Autodesk Inventor part; units mm, degrees
(part 3 of 6)
  spline S504 degree 2 poles (-98.2003, 62.4281) (-98.3407, 62.5686) (-98.4987, 62.6915) knots 0 0 0 1 1 1
  spline S505 degree 2 poles (-71.4426, 63.5518) (-71.4426, 63.9557) (-70.8807, 64.5) (-70.4944, 64.5) knots 0 0 0 1 2 2 2
  spline S506 degree 2 poles (-70.4944, 64.5) (-70.0906, 64.5) (-69.5287, 63.9557) (-69.5287, 63.5518) knots 0 0 0 1 2 2 2
  line L659 (-69.5287, 63.5518) -> (-69.5287, 54.9657)
  line L660 (-69.5287, 54.9657) -> (-63.8222, 54.9657)
  line L661 (-63.8222, 54.9657) -> (-63.8222, 63.5518)
  spline S507 degree 2 poles (-63.8222, 63.5518) (-63.8222, 63.9557) (-63.2603, 64.5) (-62.8565, 64.5) knots 0 0 0 1 2 2 2
  spline S508 degree 2 poles (-62.8565, 64.5) (-62.4702, 64.5) (-61.9083, 63.9557) (-61.9083, 63.5518) knots 0 0 0 1 2 2 2
  line L662 (-61.9083, 63.5518) -> (-61.9083, 44.4482)
  spline S509 degree 2 poles (-61.9083, 44.4482) (-61.9083, 44.0619) (-62.4702, 43.5) (-62.8565, 43.5) knots 0 0 0 1 2 2 2
  spline S510 degree 2 poles (-62.8565, 43.5) (-63.2603, 43.5) (-63.8222, 44.0619) (-63.8222, 44.4482) knots 0 0 0 1 2 2 2
  line L663 (-63.8222, 44.4482) -> (-63.8222, 53.0518)
  line L664 (-63.8222, 53.0518) -> (-69.5287, 53.0518)
  line L665 (-69.5287, 53.0518) -> (-69.5287, 44.4482)
  spline S511 degree 2 poles (-69.5287, 44.4482) (-69.5287, 44.0619) (-70.0906, 43.5) (-70.4944, 43.5) knots 0 0 0 1 2 2 2
  spline S512 degree 2 poles (-70.4944, 43.5) (-70.8807, 43.5) (-71.4426, 44.0619) (-71.4426, 44.4482) knots 0 0 0 1 2 2 2
  line L666 (-71.4426, 44.4482) -> (-71.4426, 63.5518)
  spline S513 degree 2 poles (-33.3246, 49.8211) (-32.9383, 49.8211) (-32.3764, 49.2592) (-32.3764, 48.8554) knots 0 0 0 1 2 2 2
  spline S514 degree 2 poles (-32.3764, 48.8554) (-32.3764, 48.4691) (-32.9383, 47.9072) (-33.3246, 47.9072) knots 0 0 0 1 2 2 2
  line L667 (-33.3246, 47.9072) -> (-36.5026, 47.9072)
  line L668 (-36.5026, 47.9072) -> (-37.4684, 44.2901)
  spline S515 degree 2 poles (-37.4684, 44.2901) (-37.5562, 43.9916) (-37.7493, 43.7809) knots 0 0 0 1 1 1
  spline S516 degree 2 poles (-37.7493, 43.7809) (-38.0302, 43.5) (-38.4165, 43.5) knots 0 0 0 1 1 1
  spline S517 degree 2 poles (-38.4165, 43.5) (-38.8204, 43.5) (-39.3822, 44.0619) (-39.3822, 44.4482) knots 0 0 0 1 2 2 2
  spline S518 degree 2 poles (-39.3822, 44.4482) (-39.3822, 44.5711) (-39.3647, 44.6589) knots 0 0 0 1 1 1
  line L669 (-39.3647, 44.6589) -> (-34.2727, 63.6572)
  spline S519 degree 2 poles (-34.2727, 63.6572) (-34.2025, 63.9732) (-33.9918, 64.2015) knots 0 0 0 1 1 1
  spline S520 degree 2 poles (-33.9918, 64.2015) (-33.7108, 64.5) (-33.3246, 64.5) knots 0 0 0 1 1 1
  spline S521 degree 2 poles (-33.3246, 64.5) (-32.9383, 64.5) (-32.6398, 64.2015) knots 0 0 0 1 1 1
  spline S522 degree 2 poles (-32.6398, 64.2015) (-32.4642, 63.9732) (-32.394, 63.6572) knots 0 0 0 1 1 1
  line L670 (-32.394, 63.6572) -> (-27.302, 44.6589)
  spline S523 degree 2 poles (-27.302, 44.6589) (-27.2844, 44.5711) (-27.2844, 44.4482) knots 0 0 0 1 1 1
  spline S524 degree 2 poles (-27.2844, 44.4482) (-27.2844, 44.0619) (-27.8463, 43.5) (-28.2326, 43.5) knots 0 0 0 1 2 2 2
  spline S525 degree 2 poles (-28.2326, 43.5) (-28.6364, 43.5) (-28.8998, 43.7809) knots 0 0 0 1 1 1
  spline S526 degree 2 poles (-28.8998, 43.7809) (-29.1105, 43.9916) (-29.1983, 44.2901) knots 0 0 0 1 1 1
  line L671 (-29.1983, 44.2901) -> (-33.3246, 59.7943)
  line L672 (-33.3246, 59.7943) -> (-35.9935, 49.8211)
  line L673 (-35.9935, 49.8211) -> (-33.3246, 49.8211)
  spline S527 degree 2 poles (-4.4511, 63.8503) (-4.4511, 64.2542) (-3.8892, 64.8161) (-3.5029, 64.8161) knots 0 0 0 1 2 2 2
  spline S528 degree 2 poles (-3.5029, 64.8161) (-3.0991, 64.8161) (-2.5372, 64.2542) (-2.5372, 63.8503) knots 0 0 0 1 2 2 2
  line L674 (-2.5372, 63.8503) -> (-2.5372, 47.9599)
  spline S529 degree 2 poles (-2.5372, 47.9599) (-2.5372, 46.9064) (-1.0447, 45.4139) (0.0088, 45.4139) knots 0 0 0 1 2 2 2
  spline S530 degree 2 poles (0.0088, 45.4139) (1.0623, 45.4139) (2.5548, 46.9064) (2.5548, 47.9599) knots 0 0 0 1 2 2 2
  line L675 (2.5548, 47.9599) -> (2.5548, 63.8503)
  spline S531 degree 2 poles (2.5548, 63.8503) (2.5548, 64.2542) (3.0991, 64.8161) (3.5029, 64.8161) knots 0 0 0 1 2 2 2
  spline S532 degree 2 poles (3.5029, 64.8161) (3.9068, 64.8161) (4.4686, 64.2542) (4.4686, 63.8503) knots 0 0 0 1 2 2 2
  line L676 (4.4686, 63.8503) -> (4.4686, 47.9599)
  spline S533 degree 2 poles (4.4686, 47.9599) (4.4686, 46.1162) (1.8524, 43.5) (0.0088, 43.5) knots 0 0 0 1 2 2 2
  spline S534 degree 2 poles (0.0088, 43.5) (-1.8349, 43.5) (-4.4511, 46.1162) (-4.4511, 47.9599) knots 0 0 0 1 2 2 2
  line L677 (-4.4511, 47.9599) -> (-4.4511, 63.8503)
  spline S535 degree 2 poles (38.118, 47.9423) (38.118, 46.0987) (36.8011, 44.7993) knots 0 0 0 1 1 1
  spline S536 degree 2 poles (36.8011, 44.7993) (35.6423, 43.6054) (34.0445, 43.5) knots 0 0 0 1 1 1
  spline S537 degree 2 poles (34.0445, 43.5) (33.5704, 43.5) (33.0261, 44.0619) (33.0261, 44.4482) knots 0 0 0 1 2 2 2
  spline S538 degree 2 poles (33.0261, 44.4482) (33.0261, 44.852) (33.307, 45.1329) knots 0 0 0 1 1 1
  spline S539 degree 2 poles (33.307, 45.1329) (33.5353, 45.3788) (33.8864, 45.4139) knots 0 0 0 1 1 1
  spline S540 degree 2 poles (33.8864, 45.4139) (34.7995, 45.4841) (35.4491, 46.1513) knots 0 0 0 1 1 1
  spline S541 degree 2 poles (35.4491, 46.1513) (36.2042, 46.8888) (36.2042, 47.9423) knots 0 0 0 1 1 1
  line L678 (36.2042, 47.9423) -> (36.2042, 50.5585)
  spline S542 degree 2 poles (36.2042, 50.5585) (36.2042, 51.5945) (35.4491, 52.3495) knots 0 0 0 1 1 1
  spline S543 degree 2 poles (35.4491, 52.3495) (34.8521, 52.964) (34.0445, 53.0694) knots 0 0 0 1 1 1
  spline S544 degree 2 poles (34.0445, 53.0694) (33.5704, 53.0694) (33.307, 53.3503) knots 0 0 0 1 1 1
  spline S545 degree 2 poles (33.307, 53.3503) (33.0261, 53.6313) (33.0261, 54.0176) knots 0 0 0 1 1 1
  line L679 (33.0261, 54.0176) -> (33.0261, 54.0351)
  spline S546 degree 2 poles (33.0261, 54.0351) (33.0261, 54.439) (33.307, 54.7199) knots 0 0 0 1 1 1
  spline S547 degree 2 poles (33.307, 54.7199) (33.5704, 55.0008) (34.0445, 55.0008) knots 0 0 0 1 1 1
  spline S548 degree 2 poles (34.0445, 55.0008) (34.8521, 55.1062) (35.4491, 55.7032) knots 0 0 0 1 1 1
  spline S549 degree 2 poles (35.4491, 55.7032) (36.2042, 56.4582) (36.2042, 57.5117) knots 0 0 0 1 1 1
  line L680 (36.2042, 57.5117) -> (36.2042, 60.0928)
  spline S550 degree 2 poles (36.2042, 60.0928) (36.2042, 61.1288) (35.4491, 61.8838) knots 0 0 0 1 1 1
  spline S551 degree 2 poles (35.4491, 61.8838) (34.7995, 62.5334) (33.8864, 62.6212) knots 0 0 0 1 1 1
  spline S552 degree 2 poles (33.8864, 62.6212) (33.5353, 62.6564) (33.307, 62.9022) knots 0 0 0 1 1 1
  spline S553 degree 2 poles (33.307, 62.9022) (33.0261, 63.1656) (33.0261, 63.5694) knots 0 0 0 1 1 1
  spline S554 degree 2 poles (33.0261, 63.5694) (33.0261, 63.9732) (33.5704, 64.5176) (34.0445, 64.5176) knots 0 0 0 1 2 2 2
  spline S555 degree 2 poles (34.0445, 64.5176) (35.6423, 64.4122) (36.8011, 63.2358) knots 0 0 0 1 1 1
  spline S556 degree 2 poles (36.8011, 63.2358) (38.118, 61.9365) (38.118, 60.0928) knots 0 0 0 1 1 1
  line L681 (38.118, 60.0928) -> (38.118, 57.5117)
  spline S557 degree 2 poles (38.118, 57.5117) (38.118, 55.3344) (36.45, 54.0176) knots 0 0 0 1 1 1
  spline S558 degree 2 poles (36.45, 54.0176) (38.118, 52.7182) (38.118, 50.5585) knots 0 0 0 1 1 1
  line L682 (38.118, 50.5585) -> (38.118, 47.9423)
  spline S559 degree 2 poles (29.1983, 63.5694) (29.1983, 63.9732) (29.7602, 64.5176) (30.1465, 64.5176) knots 0 0 0 1 2 2 2
  spline S560 degree 2 poles (30.1465, 64.5176) (30.5503, 64.5176) (31.1122, 63.9732) (31.1122, 63.5694) knots 0 0 0 1 2 2 2
  line L683 (31.1122, 63.5694) -> (31.1122, 44.4657)
  spline S561 degree 2 poles (31.1122, 44.4657) (31.1122, 44.0794) (30.5503, 43.5176) (30.1465, 43.5176) knots 0 0 0 1 2 2 2
  spline S562 degree 2 poles (30.1465, 43.5176) (29.7602, 43.5176) (29.1983, 44.0794) (29.1983, 44.4657) knots 0 0 0 1 2 2 2
  line L684 (29.1983, 44.4657) -> (29.1983, 63.5694)
  spline S563 degree 2 poles (65.7097, 63.5518) (65.7097, 63.9557) (66.2716, 64.5) (66.6579, 64.5) knots 0 0 0 1 2 2 2
  spline S564 degree 2 poles (66.6579, 64.5) (67.0617, 64.5) (67.6236, 63.9557) (67.6236, 63.5518) knots 0 0 0 1 2 2 2
  line L685 (67.6236, 63.5518) -> (67.6236, 44.4482)
  spline S565 degree 2 poles (67.6236, 44.4482) (67.6236, 44.0619) (67.0617, 43.5) (66.6579, 43.5) knots 0 0 0 1 2 2 2
  spline S566 degree 2 poles (66.6579, 43.5) (66.2716, 43.5) (65.7097, 44.0619) (65.7097, 44.4482) knots 0 0 0 1 2 2 2
  line L686 (65.7097, 44.4482) -> (65.7097, 63.5518)
  spline S567 degree 2 poles (96.8219, 63.5518) (96.8219, 63.9557) (97.3838, 64.5) (97.7701, 64.5) knots 0 0 0 1 2 2 2
  line L687 (97.7701, 64.5) -> (103.8453, 64.5)
  spline S568 degree 2 poles (103.8453, 64.5) (104.2316, 64.5) (104.7935, 63.9557) (104.7935, 63.5518) knots 0 0 0 1 2 2 2
  spline S569 degree 2 poles (104.7935, 63.5518) (104.7935, 63.1656) (104.2316, 62.6037) (103.8453, 62.6037) knots 0 0 0 1 2 2 2
  line L688 (103.8453, 62.6037) -> (98.7358, 62.6037)
  line L689 (98.7358, 62.6037) -> (98.7358, 54.9657)
  line L690 (98.7358, 54.9657) -> (102.862, 54.9657)
  spline S570 degree 2 poles (102.862, 54.9657) (103.2659, 54.9657) (103.8278, 54.4038) (103.8278, 54) knots 0 0 0 1 2 2 2
  spline S571 degree 2 poles (103.8278, 54) (103.8278, 53.6137) (103.2659, 53.0518) (102.862, 53.0518) knots 0 0 0 1 2 2 2
  line L691 (102.862, 53.0518) -> (98.7358, 53.0518)
  line L692 (98.7358, 53.0518) -> (98.7358, 45.4139)
  line L693 (98.7358, 45.4139) -> (103.8453, 45.4139)
  spline S572 degree 2 poles (103.8453, 45.4139) (104.2316, 45.4139) (104.7935, 44.852) (104.7935, 44.4482) knots 0 0 0 1 2 2 2
  spline S573 degree 2 poles (104.7935, 44.4482) (104.7935, 44.0794) (104.2316, 43.5) (103.8453, 43.5) knots 0 0 0 1 2 2 2
  line L694 (103.8453, 43.5) -> (97.7701, 43.5)
  spline S574 degree 2 poles (97.7701, 43.5) (97.3838, 43.5) (96.8219, 44.0619) (96.8219, 44.4482) knots 0 0 0 1 2 2 2
  line L695 (96.8219, 44.4482) -> (96.8219, 63.5518)
  spline S575 degree 2 poles (136.529, 63.4816) (136.7924, 63.1831) (136.7924, 62.8144) knots 0 0 0 1 1 1
  spline S576 degree 2 poles (136.7924, 62.8144) (136.7924, 62.4105) (136.2305, 61.8487) (135.8442, 61.8487) knots 0 0 0 1 2 2 2
  spline S577 degree 2 poles (135.8442, 61.8487) (135.4404, 61.8487) (135.177, 62.1296) knots 0 0 0 1 1 1
  spline S578 degree 2 poles (135.177, 62.1296) (134.3693, 62.9197) (133.3333, 62.9197) knots 0 0 0 1 1 1
  spline S579 degree 2 poles (133.3333, 62.9197) (132.2623, 62.9197) (130.7873, 61.4273) (130.7873, 60.3737) knots 0 0 0 1 2 2 2
  line L696 (130.7873, 60.3737) -> (130.7873, 47.9599)
  spline S580 degree 2 poles (130.7873, 47.9599) (130.7873, 46.9064) (132.2623, 45.4139) (133.3333, 45.4139) knots 0 0 0 1 2 2 2
  line L697 (133.3333, 45.4139) -> (135.8793, 45.4139)
  line L698 (135.8793, 45.4139) -> (135.8793, 52.7358)
  line L699 (135.8793, 52.7358) -> (134.9136, 52.7358)
  spline S581 degree 2 poles (134.9136, 52.7358) (134.5273, 52.7358) (133.9654, 53.2977) (133.9654, 53.6839) knots 0 0 0 1 2 2 2
  spline S582 degree 2 poles (133.9654, 53.6839) (133.9654, 54.0878) (134.5273, 54.6497) (134.9136, 54.6497) knots 0 0 0 1 2 2 2
  line L700 (134.9136, 54.6497) -> (136.845, 54.6497)
  spline S583 degree 2 poles (136.845, 54.6497) (137.2489, 54.6497) (137.7756, 54.0878) (137.7756, 53.6839) knots 0 0 0 1 2 2 2
  line L701 (137.7756, 53.6839) -> (137.7756, 44.4482)
  spline S584 degree 2 poles (137.7756, 44.4482) (137.7756, 44.0794) (137.2313, 43.5) (136.8275, 43.5) knots 0 0 0 1 2 2 2
  line L702 (136.8275, 43.5) -> (133.3333, 43.5)
  spline S585 degree 2 poles (133.3333, 43.5) (131.4721, 43.5) (128.8735, 46.0987) (128.8735, 47.9423) knots 0 0 0 1 2 2 2
  line L703 (128.8735, 47.9423) -> (128.8735, 60.3913)
  spline S586 degree 2 poles (128.8735, 60.3913) (128.8735, 62.2349) (131.4721, 64.8512) (133.3333, 64.8512) knots 0 0 0 1 2 2 2
  spline S587 degree 2 poles (133.3333, 64.8512) (135.177, 64.8512) (136.529, 63.4816) knots 0 0 0 1 1 1
  spline S588 degree 2 poles (163.4886, 63.5518) (163.4886, 63.9557) (164.0504, 64.5) (164.4367, 64.5) knots 0 0 0 1 2 2 2
  line L704 (164.4367, 64.5) -> (170.512, 64.5)
  spline S589 degree 2 poles (170.512, 64.5) (170.8983, 64.5) (171.4601, 63.9557) (171.4601, 63.5518) knots 0 0 0 1 2 2 2
  spline S590 degree 2 poles (171.4601, 63.5518) (171.4601, 63.1656) (170.8983, 62.6037) (170.512, 62.6037) knots 0 0 0 1 2 2 2
  line L705 (170.512, 62.6037) -> (165.4025, 62.6037)
  line L706 (165.4025, 62.6037) -> (165.4025, 54.9657)
  line L707 (165.4025, 54.9657) -> (169.5287, 54.9657)
  spline S591 degree 2 poles (169.5287, 54.9657) (169.9326, 54.9657) (170.4944, 54.4038) (170.4944, 54) knots 0 0 0 1 2 2 2
  spline S592 degree 2 poles (170.4944, 54) (170.4944, 53.6137) (169.9326, 53.0518) (169.5287, 53.0518) knots 0 0 0 1 2 2 2
  line L708 (169.5287, 53.0518) -> (165.4025, 53.0518)
  line L709 (165.4025, 53.0518) -> (165.4025, 45.4139)
  line L710 (165.4025, 45.4139) -> (170.512, 45.4139)
  spline S593 degree 2 poles (170.512, 45.4139) (170.8983, 45.4139) (171.4601, 44.852) (171.4601, 44.4482) knots 0 0 0 1 2 2 2
  spline S594 degree 2 poles (171.4601, 44.4482) (171.4601, 44.0794) (170.8983, 43.5) (170.512, 43.5) knots 0 0 0 1 2 2 2
  line L711 (170.512, 43.5) -> (164.4367, 43.5)
  spline S595 degree 2 poles (164.4367, 43.5) (164.0504, 43.5) (163.4886, 44.0619) (163.4886, 44.4482) knots 0 0 0 1 2 2 2
  line L712 (163.4886, 44.4482) -> (163.4886, 63.5518)
  spline S596 degree 2 poles (-172.698, -8.6589) (-172.7156, -8.5535) (-172.7156, -8.4482) knots 0 0 0 1 1 1
  spline S597 degree 2 poles (-172.7156, -8.4482) (-172.7156, -8.0443) (-172.1537, -7.5) (-171.7499, -7.5) knots 0 0 0 1 2 2 2
  spline S598 degree 2 poles (-171.7499, -7.5) (-171.3636, -7.5) (-171.0826, -7.7634) knots 0 0 0 1 1 1
  spline S599 degree 2 poles (-171.0826, -7.7634) (-170.8719, -7.9916) (-170.8017, -8.2901) knots 0 0 0 1 1 1
  line L713 (-170.8017, -8.2901) -> (-166.6579, -23.8119)
  line L714 (-166.6579, -23.8119) -> (-162.5316, -8.2901)
  spline S600 degree 2 poles (-162.5316, -8.2901) (-162.4614, -7.9916) (-162.2331, -7.7634) knots 0 0 0 1 1 1
  spline S601 degree 2 poles (-162.2331, -7.7634) (-161.9698, -7.5) (-161.5659, -7.5) knots 0 0 0 1 1 1
  spline S602 degree 2 poles (-161.5659, -7.5) (-161.1796, -7.5) (-160.6178, -8.0443) (-160.6178, -8.4482) knots 0 0 0 1 2 2 2
  spline S603 degree 2 poles (-160.6178, -8.4482) (-160.6178, -8.5535) (-160.6353, -8.6589) knots 0 0 0 1 1 1
  line L715 (-160.6353, -8.6589) -> (-165.7273, -27.6747)
  spline S604 degree 2 poles (-165.7273, -27.6747) (-165.7975, -27.9732) (-165.9731, -28.2191) knots 0 0 0 1 1 1
  spline S605 degree 2 poles (-165.9731, -28.2191) (-166.2716, -28.5) (-166.6579, -28.5) knots 0 0 0 1 1 1
  spline S606 degree 2 poles (-166.6579, -28.5) (-167.0442, -28.5) (-167.3251, -28.2191) knots 0 0 0 1 1 1
  spline S607 degree 2 poles (-167.3251, -28.2191) (-167.5358, -27.9732) (-167.606, -27.6747) knots 0 0 0 1 1 1
  line L716 (-167.606, -27.6747) -> (-172.698, -8.6589)
  spline S608 degree 2 poles (-134.2903, -8.4482) (-134.2903, -8.0443) (-133.7284, -7.5) (-133.3421, -7.5) knots 0 0 0 1 2 2 2
  spline S609 degree 2 poles (-133.3421, -7.5) (-132.9383, -7.5) (-132.3764, -8.0443) (-132.3764, -8.4482) knots 0 0 0 1 2 2 2
  line L717 (-132.3764, -8.4482) -> (-132.3764, -27.5518)
  spline S610 degree 2 poles (-132.3764, -27.5518) (-132.3764, -27.9381) (-132.9383, -28.5) (-133.3421, -28.5) knots 0 0 0 1 2 2 2
  spline S611 degree 2 poles (-133.3421, -28.5) (-133.7284, -28.5) (-134.2903, -27.9381) (-134.2903, -27.5518) knots 0 0 0 1 2 2 2
  line L718 (-134.2903, -27.5518) -> (-134.2903, -8.4482)
  spline S612 degree 2 poles (-103.1781, -8.4482) (-103.1781, -8.0443) (-102.6162, -7.5) (-102.2299, -7.5) knots 0 0 0 1 2 2 2
  line L719 (-102.2299, -7.5) -> (-96.1547, -7.5)
  spline S613 degree 2 poles (-96.1547, -7.5) (-95.7684, -7.5) (-95.2065, -8.0443) (-95.2065, -8.4482) knots 0 0 0 1 2 2 2
  spline S614 degree 2 poles (-95.2065, -8.4482) (-95.2065, -8.8344) (-95.7684, -9.3963) (-96.1547, -9.3963) knots 0 0 0 1 2 2 2
  line L720 (-96.1547, -9.3963) -> (-101.2642, -9.3963)
  line L721 (-101.2642, -9.3963) -> (-101.2642, -17.0343)
  line L722 (-101.2642, -17.0343) -> (-97.138, -17.0343)
  spline S615 degree 2 poles (-97.138, -17.0343) (-96.7341, -17.0343) (-96.1722, -17.5962) (-96.1722, -18) knots 0 0 0 1 2 2 2
  spline S616 degree 2 poles (-96.1722, -18) (-96.1722, -18.3863) (-96.7341, -18.9482) (-97.138, -18.9482) knots 0 0 0 1 2 2 2
  line L723 (-97.138, -18.9482) -> (-101.2642, -18.9482)
  line L724 (-101.2642, -18.9482) -> (-101.2642, -26.5861)
  line L725 (-101.2642, -26.5861) -> (-96.1547, -26.5861)
  spline S617 degree 2 poles (-96.1547, -26.5861) (-95.7684, -26.5861) (-95.2065, -27.148) (-95.2065, -27.5518) knots 0 0 0 1 2 2 2
  spline S618 degree 2 poles (-95.2065, -27.5518) (-95.2065, -27.9206) (-95.7684, -28.5) (-96.1547, -28.5) knots 0 0 0 1 2 2 2
  line L726 (-96.1547, -28.5) -> (-102.2299, -28.5)
  spline S619 degree 2 poles (-102.2299, -28.5) (-102.6162, -28.5) (-103.1781, -27.9381) (-103.1781, -27.5518) knots 0 0 0 1 2 2 2
  line L727 (-103.1781, -27.5518) -> (-103.1781, -8.4482)
  spline S620 degree 2 poles (-65.183, -19.8436) (-64.744, -19.7207) (-64.3577, -19.352) knots 0 0 0 1 1 1
  spline S621 degree 2 poles (-64.3577, -19.352) (-63.7958, -18.7901) (-63.7958, -18) knots 0 0 0 1 1 1
  line L728 (-63.7958, -18) -> (-63.7958, -11.3102)
  spline S622 degree 2 poles (-63.7958, -11.3102) (-63.7958, -10.5201) (-64.9196, -9.3963) (-65.7097, -9.3963) knots 0 0 0 1 2 2 2
  line L729 (-65.7097, -9.3963) -> (-68.8878, -9.3963)
  line L730 (-68.8878, -9.3963) -> (-68.8878, -27.5518)
  spline S623 degree 2 poles (-68.8878, -27.5518) (-68.8878, -27.9381) (-69.4497, -28.5) (-69.8535, -28.5) knots 0 0 0 1 2 2 2
  spline S624 degree 2 poles (-69.8535, -28.5) (-70.2398, -28.5) (-70.8017, -27.9381) (-70.8017, -27.5518) knots 0 0 0 1 2 2 2
  line L731 (-70.8017, -27.5518) -> (-70.8017, -8.4482)
  spline S625 degree 2 poles (-70.8017, -8.4482) (-70.8017, -8.0443) (-70.2398, -7.5) (-69.8535, -7.5) knots 0 0 0 1 2 2 2
  line L732 (-69.8535, -7.5) -> (-65.7097, -7.5)
  spline S626 degree 2 poles (-65.7097, -7.5) (-64.1295, -7.5) (-61.882, -9.7299) (-61.882, -11.3102) knots 0 0 0 1 2 2 2
  line L733 (-61.882, -11.3102) -> (-61.882, -18)
  spline S627 degree 2 poles (-61.882, -18) (-61.882, -19.5627) (-63.0057, -20.6865) knots 0 0 0 1 1 1
  spline S628 degree 2 poles (-63.0057, -20.6865) (-63.3569, -21.0376) (-63.7432, -21.2659) knots 0 0 0 1 1 1
  line L734 (-63.7432, -21.2659) -> (-61.3552, -27.1304)
  spline S629 degree 2 poles (-61.3552, -27.1304) (-61.2499, -27.3411) (-61.2499, -27.5518) knots 0 0 0 1 1 1
  spline S630 degree 2 poles (-61.2499, -27.5518) (-61.2499, -27.6923) (-61.3025, -27.8328) knots 0 0 0 1 1 1
  spline S631 degree 2 poles (-61.3025, -27.8328) (-61.4254, -28.2191) (-61.7766, -28.3946) knots 0 0 0 1 1 1
  spline S632 degree 2 poles (-61.7766, -28.3946) (-61.9873, -28.5) (-62.198, -28.5) knots 0 0 0 1 1 1
  spline S633 degree 2 poles (-62.198, -28.5) (-62.356, -28.5) (-62.4965, -28.4649) knots 0 0 0 1 1 1
  spline S634 degree 2 poles (-62.4965, -28.4649) (-62.8828, -28.342) (-63.0584, -27.9732) knots 0 0 0 1 1 1
  line L735 (-63.0584, -27.9732) -> (-65.78, -21.2308)
  spline S635 degree 2 poles (-65.78, -21.2308) (-65.9029, -21.0201) (-65.9029, -20.7567) knots 0 0 0 1 1 1
  spline S636 degree 2 poles (-65.9029, -20.7567) (-65.9029, -20.3704) (-65.6044, -20.0719) knots 0 0 0 1 1 1
  spline S637 degree 2 poles (-65.6044, -20.0719) (-65.4288, -19.8963) (-65.183, -19.8436) knots 0 0 0 1 1 1
  spline S638 degree 2 poles (-34.2903, -8.4482) (-34.2903, -8.0443) (-33.7284, -7.5) (-33.3421, -7.5) knots 0 0 0 1 2 2 2
  spline S639 degree 2 poles (-33.3421, -7.5) (-32.9383, -7.5) (-32.3764, -8.0443) (-32.3764, -8.4482) knots 0 0 0 1 2 2 2
  line L736 (-32.3764, -8.4482) -> (-32.3764, -27.5518)
  spline S640 degree 2 poles (-32.3764, -27.5518) (-32.3764, -27.9381) (-32.9383, -28.5) (-33.3421, -28.5) knots 0 0 0 1 2 2 2
  spline S641 degree 2 poles (-33.3421, -28.5) (-33.7284, -28.5) (-34.2903, -27.9381) (-34.2903, -27.5518) knots 0 0 0 1 2 2 2
  line L737 (-34.2903, -27.5518) -> (-34.2903, -8.4482)
  spline S642 degree 2 poles (3.1781, -17.0343) (3.5819, -17.0343) (4.1438, -17.5962) (4.1438, -18) knots 0 0 0 1 2 2 2
  spline S643 degree 2 poles (4.1438, -18) (4.1438, -18.3863) (3.5819, -18.9482) (3.1781, -18.9482) knots 0 0 0 1 2 2 2
  line L738 (3.1781, -18.9482) -> (-0.9482, -18.9482)
  line L739 (-0.9482, -18.9482) -> (-0.9482, -27.5518)
  spline S644 degree 2 poles (-0.9482, -27.5518) (-0.9482, -27.9381) (-1.51, -28.5) (-1.9139, -28.5) knots 0 0 0 1 2 2 2
  spline S645 degree 2 poles (-1.9139, -28.5) (-2.3002, -28.5) (-2.862, -27.9381) (-2.862, -27.5518) knots 0 0 0 1 2 2 2
  line L740 (-2.862, -27.5518) -> (-2.862, -8.4482)
  spline S646 degree 2 poles (-2.862, -8.4482) (-2.862, -8.0443) (-2.3002, -7.5) (-1.9139, -7.5) knots 0 0 0 1 2 2 2
  line L741 (-1.9139, -7.5) -> (4.1614, -7.5)
  spline S647 degree 2 poles (4.1614, -7.5) (4.5477, -7.5) (5.1095, -8.0443) (5.1095, -8.4482) knots 0 0 0 1 2 2 2
  spline S648 degree 2 poles (5.1095, -8.4482) (5.1095, -8.8344) (4.5477, -9.3963) (4.1614, -9.3963) knots 0 0 0 1 2 2 2
  line L742 (4.1614, -9.3963) -> (-0.9482, -9.3963)
  line L743 (-0.9482, -9.3963) -> (-0.9482, -17.0343)
  line L744 (-0.9482, -17.0343) -> (3.1781, -17.0343)
  spline S649 degree 2 poles (28.8822, -8.1497) (28.8822, -7.7458) (29.4441, -7.1839) (29.8304, -7.1839) knots 0 0 0 1 2 2 2
  spline S650 degree 2 poles (29.8304, -7.1839) (30.2343, -7.1839) (30.7961, -7.7458) (30.7961, -8.1497) knots 0 0 0 1 2 2 2
  line L745 (30.7961, -8.1497) -> (30.7961, -24.0401)
  spline S651 degree 2 poles (30.7961, -24.0401) (30.7961, -25.0936) (32.2886, -26.5861) (33.3421, -26.5861) knots 0 0 0 1 2 2 2
  spline S652 degree 2 poles (33.3421, -26.5861) (34.3956, -26.5861) (35.8881, -25.0936) (35.8881, -24.0401) knots 0 0 0 1 2 2 2
  line L746 (35.8881, -24.0401) -> (35.8881, -8.1497)
  spline S653 degree 2 poles (35.8881, -8.1497) (35.8881, -7.7458) (36.4324, -7.1839) (36.8363, -7.1839) knots 0 0 0 1 2 2 2
  spline S654 degree 2 poles (36.8363, -7.1839) (37.2401, -7.1839) (37.802, -7.7458) (37.802, -8.1497) knots 0 0 0 1 2 2 2
  line L747 (37.802, -8.1497) -> (37.802, -24.0401)
  spline S655 degree 2 poles (37.802, -24.0401) (37.802, -25.8838) (35.1858, -28.5) (33.3421, -28.5) knots 0 0 0 1 2 2 2
  spline S656 degree 2 poles (33.3421, -28.5) (31.4985, -28.5) (28.8822, -25.8838) (28.8822, -24.0401) knots 0 0 0 1 2 2 2
  line L748 (28.8822, -24.0401) -> (28.8822, -8.1497)
  spline S657 degree 2 poles (31.0244, -2.0744) (31.5511, -2.0744) (32.3062, -2.8294) (32.3062, -3.3562) knots 0 0 0 1 2 2 2
  spline S658 degree 2 poles (32.3062, -3.3562) (32.3062, -3.8829) (31.5511, -4.6204) (31.0244, -4.6204) knots 0 0 0 1 2 2 2
  spline S659 degree 2 poles (31.0244, -4.6204) (30.4976, -4.6204) (29.7602, -3.8829) (29.7602, -3.3562) knots 0 0 0 1 2 2 2
  spline S660 degree 2 poles (29.7602, -3.3562) (29.7602, -2.8294) (30.4976, -2.0744) (31.0244, -2.0744) knots 0 0 0 1 2 2 2
  spline S661 degree 2 poles (35.6598, -2.0744) (36.1866, -2.0744) (36.9416, -2.8294) (36.9416, -3.3562) knots 0 0 0 1 2 2 2
  spline S662 degree 2 poles (36.9416, -3.3562) (36.9416, -3.8829) (36.1866, -4.6204) (35.6598, -4.6204) knots 0 0 0 1 2 2 2
  spline S663 degree 2 poles (35.6598, -4.6204) (35.1331, -4.6204) (34.3956, -3.8829) (34.3956, -3.3562) knots 0 0 0 1 2 2 2
  spline S664 degree 2 poles (34.3956, -3.3562) (34.3956, -2.8294) (35.1331, -2.0744) (35.6598, -2.0744) knots 0 0 0 1 2 2 2
  spline S665 degree 2 poles (69.8448, -17.0343) (70.2486, -17.0343) (70.8105, -17.5962) (70.8105, -18) knots 0 0 0 1 2 2 2
  spline S666 degree 2 poles (70.8105, -18) (70.8105, -18.3863) (70.2486, -18.9482) (69.8448, -18.9482) knots 0 0 0 1 2 2 2
  line L749 (69.8448, -18.9482) -> (65.7185, -18.9482)
  line L750 (65.7185, -18.9482) -> (65.7185, -27.5518)
  spline S667 degree 2 poles (65.7185, -27.5518) (65.7185, -27.9381) (65.1566, -28.5) (64.7528, -28.5) knots 0 0 0 1 2 2 2
  spline S668 degree 2 poles (64.7528, -28.5) (64.3665, -28.5) (63.8046, -27.9381) (63.8046, -27.5518) knots 0 0 0 1 2 2 2
  line L751 (63.8046, -27.5518) -> (63.8046, -8.4482)
  spline S669 degree 2 poles (63.8046, -8.4482) (63.8046, -8.0443) (64.3665, -7.5) (64.7528, -7.5) knots 0 0 0 1 2 2 2
  line L752 (64.7528, -7.5) -> (70.828, -7.5)
  spline S670 degree 2 poles (70.828, -7.5) (71.2143, -7.5) (71.7762, -8.0443) (71.7762, -8.4482) knots 0 0 0 1 2 2 2
  spline S671 degree 2 poles (71.7762, -8.4482) (71.7762, -8.8344) (71.2143, -9.3963) (70.828, -9.3963) knots 0 0 0 1 2 2 2
  line L753 (70.828, -9.3963) -> (65.7185, -9.3963)
  line L754 (65.7185, -9.3963) -> (65.7185, -17.0343)
  line L755 (65.7185, -17.0343) -> (69.8448, -17.0343)
  spline S672 degree 2 poles (99.0431, -8.4482) (99.0431, -8.0443) (99.6049, -7.5) (99.9912, -7.5) knots 0 0 0 1 2 2 2
  spline S673 degree 2 poles (99.9912, -7.5) (100.3951, -7.5) (100.9569, -8.0443) (100.9569, -8.4482) knots 0 0 0 1 2 2 2
  line L756 (100.9569, -8.4482) -> (100.9569, -27.5518)
  spline S674 degree 2 poles (100.9569, -27.5518) (100.9569, -27.9381) (100.3951, -28.5) (99.9912, -28.5) knots 0 0 0 1 2 2 2
  spline S675 degree 2 poles (99.9912, -28.5) (99.6049, -28.5) (99.0431, -27.9381) (99.0431, -27.5518) knots 0 0 0 1 2 2 2
  line L757 (99.0431, -27.5518) -> (99.0431, -8.4482)
  spline S676 degree 2 poles (137.6791, -23.4607) (137.6264, -23.7241) (137.4332, -23.9348) knots 0 0 0 1 1 1
  spline S677 degree 2 poles (137.4332, -23.9348) (137.1348, -24.2333) (136.7485, -24.2333) knots 0 0 0 1 1 1
  spline S678 degree 2 poles (136.7485, -24.2333) (136.3446, -24.2333) (135.7827, -23.6714) (135.7827, -23.2676) knots 0 0 0 1 2 2 2
  spline S679 degree 2 poles (135.7827, -23.2676) (135.7827, -23.1622) (135.8003, -23.0393) knots 0 0 0 1 1 1
  spline S680 degree 2 poles (135.8003, -23.0393) (135.8881, -22.7408) (135.8881, -22.3896) knots 0 0 0 1 1 1
  line L758 (135.8881, -22.3896) -> (135.8881, -9.6597)
  spline S681 degree 2 poles (135.8881, -9.6597) (135.8881, -8.6062) (134.3781, -7.1137) (133.3421, -7.1137) knots 0 0 0 1 2 2 2
  spline S682 degree 2 poles (133.3421, -7.1137) (132.2886, -7.1137) (130.7961, -8.6062) (130.7961, -9.6597) knots 0 0 0 1 2 2 2
  line L759 (130.7961, -9.6597) -> (130.7961, -22.3896)
  spline S683 degree 2 poles (130.7961, -22.3896) (130.7961, -23.4431) (132.1657, -24.7249) (133.0085, -24.9356) knots 0 0 0 1 2 2 2
  line L760 (133.0085, -24.9356) -> (137.9073, -26.6388)
  spline S684 degree 2 poles (137.9073, -26.6388) (138.2761, -26.7793) (138.4516, -27.1304) knots 0 0 0 1 1 1
  spline S685 degree 2 poles (138.4516, -27.1304) (138.557, -27.3411) (138.557, -27.5518) knots 0 0 0 1 1 1
  spline S686 degree 2 poles (138.557, -27.5518) (138.557, -27.6923) (138.5043, -27.8503) knots 0 0 0 1 1 1
  spline S687 degree 2 poles (138.5043, -27.8503) (138.3814, -28.2366) (138.0302, -28.4122) knots 0 0 0 1 1 1
  spline S688 degree 2 poles (138.0302, -28.4122) (137.802, -28.5) (137.6088, -28.5) knots 0 0 0 1 1 1
  spline S689 degree 2 poles (137.6088, -28.5) (137.4332, -28.5) (137.2752, -28.4649) knots 0 0 0 1 1 1
  line L761 (137.2752, -28.4649) -> (132.1657, -26.709)
  spline S690 degree 2 poles (132.1657, -26.709) (130.9542, -26.2701) (130.1816, -25.5502) knots 0 0 0 1 1 1
  spline S691 degree 2 poles (130.1816, -25.5502) (128.8822, -24.2333) (128.8822, -22.3896) knots 0 0 0 1 1 1
  line L762 (128.8822, -22.3896) -> (128.8822, -9.6597)
  spline S692 degree 2 poles (128.8822, -9.6597) (128.8822, -7.8161) (131.4809, -5.1998) (133.3421, -5.1998) knots 0 0 0 1 2 2 2
  spline S693 degree 2 poles (133.3421, -5.1998) (135.1858, -5.1998) (137.7844, -7.8161) (137.7844, -9.6597) knots 0 0 0 1 2 2 2
  line L763 (137.7844, -9.6597) -> (137.7844, -22.3896)
  spline S694 degree 2 poles (137.7844, -22.3896) (137.7844, -22.9515) (137.6791, -23.4607) knots 0 0 0 1 1 1
  spline S695 degree 2 poles (162.9969, -9.3963) (162.6106, -9.3963) (162.0488, -8.852) (162.0488, -8.4482) knots 0 0 0 1 2 2 2
  spline S696 degree 2 poles (162.0488, -8.4482) (162.0488, -8.0443) (162.6106, -7.5) (162.9969, -7.5) knots 0 0 0 1 2 2 2
  line L764 (162.9969, -7.5) -> (170.0028, -7.5)
  spline S697 degree 2 poles (170.0028, -7.5) (170.4066, -7.5) (170.9685, -8.0443) (170.9685, -8.4482) knots 0 0 0 1 2 2 2
  spline S698 degree 2 poles (170.9685, -8.4482) (170.9685, -8.852) (170.4066, -9.3963) (170.0028, -9.3963) knots 0 0 0 1 2 2 2
  line L765 (170.0028, -9.3963) -> (167.4568, -9.3963)
  line L766 (167.4568, -9.3963) -> (167.4568, -27.5518)
  spline S699 degree 2 poles (167.4568, -27.5518) (167.4568, -27.9381) (166.9125, -28.5) (166.5086, -28.5) knots 0 0 0 1 2 2 2
  spline S700 degree 2 poles (166.5086, -28.5) (166.1048, -28.5) (165.5429, -27.9381) (165.5429, -27.5518) knots 0 0 0 1 2 2 2
  line L767 (165.5429, -27.5518) -> (165.5429, -9.3963)
  line L768 (165.5429, -9.3963) -> (162.9969, -9.3963)
  spline S701 degree 2 poles (-170.2135, -63.0251) (-170.512, -62.6739) (-170.512, -62.2701) knots 0 0 0 1 1 1
  spline S702 degree 2 poles (-170.512, -62.2701) (-170.4769, -61.8662) (-170.1959, -61.6028) knots 0 0 0 1 1 1
  spline S703 degree 2 poles (-170.1959, -61.6028) (-169.9326, -61.357) (-169.5111, -61.357) knots 0 0 0 1 1 1
  spline S704 degree 2 poles (-169.5111, -61.357) (-169.1249, -61.3921) (-168.7912, -61.7258) knots 0 0 0 1 1 1
  spline S705 degree 2 poles (-168.7912, -61.7258) (-168.0889, -62.5159) (-167.0354, -62.5686) knots 0 0 0 1 1 1
  line L769 (-167.0354, -62.5686) -> (-166.9125, -62.5686)
  spline S706 degree 2 poles (-166.9125, -62.5686) (-165.9292, -62.5686) (-165.2093, -61.9013) knots 0 0 0 1 1 1
  spline S707 degree 2 poles (-165.2093, -61.9013) (-164.4192, -61.199) (-164.3665, -60.163) knots 0 0 0 1 1 1
  line L770 (-164.3665, -60.163) -> (-164.3665, -59.9523)
  spline S708 degree 2 poles (-164.3665, -59.9523) (-164.3665, -57.3186) (-167.5622, -53.7893) knots 0 0 0 1 1 1
  spline S709 degree 2 poles (-167.5622, -53.7893) (-170.7402, -50.2776) (-170.7402, -47.3278) knots 0 0 0 1 1 1
  line L771 (-170.7402, -47.3278) -> (-170.7402, -47.0644)
  spline S710 degree 2 poles (-170.7402, -47.0644) (-170.6349, -45.2032) (-169.2653, -43.9741) knots 0 0 0 1 1 1
  spline S711 degree 2 poles (-169.2653, -43.9741) (-167.9836, -42.8328) (-166.3155, -42.8328) knots 0 0 0 1 1 1
  line L772 (-166.3155, -42.8328) -> (-166.0521, -42.8328)
  spline S712 degree 2 poles (-166.0521, -42.8328) (-164.1909, -42.9381) (-162.9794, -44.3077) knots 0 0 0 1 1 1
  spline S713 degree 2 poles (-162.9794, -44.3077) (-162.6633, -44.6589) (-162.6633, -45.0452) knots 0 0 0 1 1 1
  spline S714 degree 2 poles (-162.6633, -45.0452) (-162.6984, -45.449) (-162.9969, -45.7124) knots 0 0 0 1 1 1
  spline S715 degree 2 poles (-162.9969, -45.7124) (-163.2603, -45.9582) (-163.629, -45.9582) knots 0 0 0 1 1 1
  spline S716 degree 2 poles (-163.629, -45.9582) (-164.068, -45.9406) (-164.3665, -45.5895) knots 0 0 0 1 1 1
  spline S717 degree 2 poles (-164.3665, -45.5895) (-165.104, -44.8169) (-166.1575, -44.7642) knots 0 0 0 1 1 1
  line L773 (-166.1575, -44.7642) -> (-166.3331, -44.7642)
  spline S718 degree 2 poles (-166.3331, -44.7642) (-167.2637, -44.7642) (-167.9836, -45.3963) knots 0 0 0 1 1 1
  spline S719 degree 2 poles (-167.9836, -45.3963) (-168.7737, -46.1162) (-168.8264, -47.1697) knots 0 0 0 1 1 1
  line L774 (-168.8264, -47.1697) -> (-168.8264, -47.3102)
  spline S720 degree 2 poles (-168.8264, -47.3102) (-168.8264, -49.5226) (-165.5956, -53.0694) knots 0 0 0 1 1 1
  spline S721 degree 2 poles (-165.5956, -53.0694) (-162.4351, -56.5811) (-162.4351, -59.8997) knots 0 0 0 1 1 1
  spline S722 degree 2 poles (-162.4351, -59.8997) (-162.4351, -60.0753) (-162.4526, -60.2508) knots 0 0 0 1 1 1
  spline S723 degree 2 poles (-162.4526, -60.2508) (-162.558, -62.112) (-163.9275, -63.3587) knots 0 0 0 1 1 1
  spline S724 degree 2 poles (-163.9275, -63.3587) (-165.2093, -64.5) (-166.8949, -64.5) knots 0 0 0 1 1 1
  line L775 (-166.8949, -64.5) -> (-167.1407, -64.5)
  spline S725 degree 2 poles (-167.1407, -64.5) (-168.9844, -64.3946) (-170.2135, -63.0251) knots 0 0 0 1 1 1
  spline S726 degree 2 poles (-133.3246, -58.1789) (-132.9383, -58.1789) (-132.3764, -58.7408) (-132.3764, -59.1446) knots 0 0 0 1 2 2 2
  spline S727 degree 2 poles (-132.3764, -59.1446) (-132.3764, -59.5309) (-132.9383, -60.0928) (-133.3246, -60.0928) knots 0 0 0 1 2 2 2
  line L776 (-133.3246, -60.0928) -> (-136.5026, -60.0928)
  line L777 (-136.5026, -60.0928) -> (-137.4684, -63.7099)
  spline S728 degree 2 poles (-137.4684, -63.7099) (-137.5562, -64.0084) (-137.7493, -64.2191) knots 0 0 0 1 1 1
  spline S729 degree 2 poles (-137.7493, -64.2191) (-138.0302, -64.5) (-138.4165, -64.5) knots 0 0 0 1 1 1
  spline S730 degree 2 poles (-138.4165, -64.5) (-138.8204, -64.5) (-139.3822, -63.9381) (-139.3822, -63.5518) knots 0 0 0 1 2 2 2
  spline S731 degree 2 poles (-139.3822, -63.5518) (-139.3822, -63.4289) (-139.3647, -63.3411) knots 0 0 0 1 1 1
  line L778 (-139.3647, -63.3411) -> (-134.2727, -44.3428)
  spline S732 degree 2 poles (-134.2727, -44.3428) (-134.2025, -44.0268) (-133.9918, -43.7985) knots 0 0 0 1 1 1
  spline S733 degree 2 poles (-133.9918, -43.7985) (-133.7108, -43.5) (-133.3246, -43.5) knots 0 0 0 1 1 1
  spline S734 degree 2 poles (-133.3246, -43.5) (-132.9383, -43.5) (-132.6398, -43.7985) knots 0 0 0 1 1 1
  spline S735 degree 2 poles (-132.6398, -43.7985) (-132.4642, -44.0268) (-132.394, -44.3428) knots 0 0 0 1 1 1
  line L779 (-132.394, -44.3428) -> (-127.302, -63.3411)
  spline S736 degree 2 poles (-127.302, -63.3411) (-127.2844, -63.4289) (-127.2844, -63.5518) knots 0 0 0 1 1 1
  spline S737 degree 2 poles (-127.2844, -63.5518) (-127.2844, -63.9381) (-127.8463, -64.5) (-128.2326, -64.5) knots 0 0 0 1 2 2 2
  spline S738 degree 2 poles (-128.2326, -64.5) (-128.6364, -64.5) (-128.8998, -64.2191) knots 0 0 0 1 1 1
  spline S739 degree 2 poles (-128.8998, -64.2191) (-129.1105, -64.0084) (-129.1983, -63.7099) knots 0 0 0 1 1 1
  line L780 (-129.1983, -63.7099) -> (-133.3246, -48.2057)
  line L781 (-133.3246, -48.2057) -> (-135.9935, -58.1789)
  line L782 (-135.9935, -58.1789) -> (-133.3246, -58.1789)
  spline S740 degree 2 poles (-135.6423, -38.3905) (-135.1155, -38.3905) (-134.3605, -39.1455) (-134.3605, -39.6722) knots 0 0 0 1 2 2 2
  spline S741 degree 2 poles (-134.3605, -39.6722) (-134.3605, -40.199) (-135.1155, -40.9365) (-135.6423, -40.9365) knots 0 0 0 1 2 2 2
  spline S742 degree 2 poles (-135.6423, -40.9365) (-136.169, -40.9365) (-136.9065, -40.199) (-136.9065, -39.6722) knots 0 0 0 1 2 2 2
  spline S743 degree 2 poles (-136.9065, -39.6722) (-136.9065, -39.1455) (-136.169, -38.3905) (-135.6423, -38.3905) knots 0 0 0 1 2 2 2
  spline S744 degree 2 poles (-131.0068, -38.3905) (-130.4801, -38.3905) (-129.7426, -39.1455) (-129.7426, -39.6722) knots 0 0 0 1 2 2 2
  spline S745 degree 2 poles (-129.7426, -39.6722) (-129.7426, -40.199) (-130.4801, -40.9365) (-131.0068, -40.9365) knots 0 0 0 1 2 2 2
  spline S746 degree 2 poles (-131.0068, -40.9365) (-131.5336, -40.9365) (-132.2886, -40.199) (-132.2886, -39.6722) knots 0 0 0 1 2 2 2
  spline S747 degree 2 poles (-132.2886, -39.6722) (-132.2886, -39.1455) (-131.5336, -38.3905) (-131.0068, -38.3905) knots 0 0 0 1 2 2 2
  spline S748 degree 2 poles (-97.1906, -61.7784) (-96.9273, -61.5151) (-96.5234, -61.5151) knots 0 0 0 1 1 1
  spline S749 degree 2 poles (-96.5234, -61.5151) (-96.1371, -61.5151) (-95.5753, -62.0594) (-95.5753, -62.4632) knots 0 0 0 1 2 2 2
  spline S750 degree 2 poles (-95.5753, -62.4632) (-95.5753, -62.8495) (-95.8386, -63.1304) knots 0 0 0 1 1 1
  spline S751 degree 2 poles (-95.8386, -63.1304) (-97.1906, -64.5) (-99.0343, -64.5) knots 0 0 0 1 1 1
  spline S752 degree 2 poles (-99.0343, -64.5) (-100.8955, -64.5) (-103.4941, -61.8838) (-103.4941, -60.0401) knots 0 0 0 1 2 2 2
  line L783 (-103.4941, -60.0401) -> (-103.4941, -47.2751)
  spline S753 degree 2 poles (-103.4941, -47.2751) (-103.4941, -45.4314) (-100.8955, -42.8152) (-99.0343, -42.8152) knots 0 0 0 1 2 2 2
  spline S754 degree 2 poles (-99.0343, -42.8152) (-97.1906, -42.8152) (-95.8386, -44.1848) knots 0 0 0 1 1 1
  spline S755 degree 2 poles (-95.8386, -44.1848) (-95.5753, -44.4833) (-95.5753, -44.852) knots 0 0 0 1 1 1
  spline S756 degree 2 poles (-95.5753, -44.852) (-95.5753, -45.2559) (-96.1371, -45.8177) (-96.5234, -45.8177) knots 0 0 0 1 2 2 2
  spline S757 degree 2 poles (-96.5234, -45.8177) (-96.9273, -45.8177) (-97.1906, -45.5368) knots 0 0 0 1 1 1
  spline S758 degree 2 poles (-97.1906, -45.5368) (-97.9983, -44.7467) (-99.0343, -44.7467) knots 0 0 0 1 1 1
  spline S759 degree 2 poles (-99.0343, -44.7467) (-100.1054, -44.7467) (-101.5803, -46.2391) (-101.5803, -47.2926) knots 0 0 0 1 2 2 2
  line L784 (-101.5803, -47.2926) -> (-101.5803, -60.0226)
  spline S760 degree 2 poles (-101.5803, -60.0226) (-101.5803, -61.0761) (-100.1054, -62.5686) (-99.0343, -62.5686) knots 0 0 0 1 2 2 2
  spline S761 degree 2 poles (-99.0343, -62.5686) (-97.9983, -62.5686) (-97.1906, -61.7784) knots 0 0 0 1 1 1
  spline S762 degree 2 poles (-71.4426, -44.4482) (-71.4426, -44.0443) (-70.8807, -43.5) (-70.4944, -43.5) knots 0 0 0 1 2 2 2
  spline S763 degree 2 poles (-70.4944, -43.5) (-70.0906, -43.5) (-69.5287, -44.0443) (-69.5287, -44.4482) knots 0 0 0 1 2 2 2
  line L785 (-69.5287, -44.4482) -> (-69.5287, -53.0343)
  line L786 (-69.5287, -53.0343) -> (-63.8222, -53.0343)
  line L787 (-63.8222, -53.0343) -> (-63.8222, -44.4482)
  spline S764 degree 2 poles (-63.8222, -44.4482) (-63.8222, -44.0443) (-63.2603, -43.5) (-62.8565, -43.5) knots 0 0 0 1 2 2 2
  spline S765 degree 2 poles (-62.8565, -43.5) (-62.4702, -43.5) (-61.9083, -44.0443) (-61.9083, -44.4482) knots 0 0 0 1 2 2 2
  line L788 (-61.9083, -44.4482) -> (-61.9083, -63.5518)
  spline S766 degree 2 poles (-61.9083, -63.5518) (-61.9083, -63.9381) (-62.4702, -64.5) (-62.8565, -64.5) knots 0 0 0 1 2 2 2
  spline S767 degree 2 poles (-62.8565, -64.5) (-63.2603, -64.5) (-63.8222, -63.9381) (-63.8222, -63.5518) knots 0 0 0 1 2 2 2
  line L789 (-63.8222, -63.5518) -> (-63.8222, -54.9482)
  line L790 (-63.8222, -54.9482) -> (-69.5287, -54.9482)
  line L791 (-69.5287, -54.9482) -> (-69.5287, -63.5518)
  spline S768 degree 2 poles (-69.5287, -63.5518) (-69.5287, -63.9381) (-70.0906, -64.5) (-70.4944, -64.5) knots 0 0 0 1 2 2 2
  spline S769 degree 2 poles (-70.4944, -64.5) (-70.8807, -64.5) (-71.4426, -63.9381) (-71.4426, -63.5518) knots 0 0 0 1 2 2 2
  line L792 (-71.4426, -63.5518) -> (-71.4426, -44.4482)
  spline S770 degree 2 poles (-36.8802, -63.0251) (-37.1787, -62.6739) (-37.1787, -62.2701) knots 0 0 0 1 1 1
  spline S771 degree 2 poles (-37.1787, -62.2701) (-37.1435, -61.8662) (-36.8626, -61.6028) knots 0 0 0 1 1 1
  spline S772 degree 2 poles (-36.8626, -61.6028) (-36.5992, -61.357) (-36.1778, -61.357) knots 0 0 0 1 1 1
  spline S773 degree 2 poles (-36.1778, -61.357) (-35.7915, -61.3921) (-35.4579, -61.7258) knots 0 0 0 1 1 1
  spline S774 degree 2 poles (-35.4579, -61.7258) (-34.7556, -62.5159) (-33.7021, -62.5686) knots 0 0 0 1 1 1
  line L793 (-33.7021, -62.5686) -> (-33.5792, -62.5686)
  spline S775 degree 2 poles (-33.5792, -62.5686) (-32.5959, -62.5686) (-31.876, -61.9013) knots 0 0 0 1 1 1
  spline S776 degree 2 poles (-31.876, -61.9013) (-31.0858, -61.199) (-31.0332, -60.163) knots 0 0 0 1 1 1
  line L794 (-31.0332, -60.163) -> (-31.0332, -59.9523)
  spline S777 degree 2 poles (-31.0332, -59.9523) (-31.0332, -57.3186) (-34.2288, -53.7893) knots 0 0 0 1 1 1
  spline S778 degree 2 poles (-34.2288, -53.7893) (-37.4069, -50.2776) (-37.4069, -47.3278) knots 0 0 0 1 1 1
  line L795 (-37.4069, -47.3278) -> (-37.4069, -47.0644)
  spline S779 degree 2 poles (-37.4069, -47.0644) (-37.3016, -45.2032) (-35.932, -43.9741) knots 0 0 0 1 1 1
  spline S780 degree 2 poles (-35.932, -43.9741) (-34.6502, -42.8328) (-32.9822, -42.8328) knots 0 0 0 1 1 1
  line L796 (-32.9822, -42.8328) -> (-32.7188, -42.8328)
  spline S781 degree 2 poles (-32.7188, -42.8328) (-30.8576, -42.9381) (-29.646, -44.3077) knots 0 0 0 1 1 1
  spline S782 degree 2 poles (-29.646, -44.3077) (-29.33, -44.6589) (-29.33, -45.0452) knots 0 0 0 1 1 1
  spline S783 degree 2 poles (-29.33, -45.0452) (-29.3651, -45.449) (-29.6636, -45.7124) knots 0 0 0 1 1 1
  spline S784 degree 2 poles (-29.6636, -45.7124) (-29.927, -45.9582) (-30.2957, -45.9582) knots 0 0 0 1 1 1
  spline S785 degree 2 poles (-30.2957, -45.9582) (-30.7347, -45.9406) (-31.0332, -45.5895) knots 0 0 0 1 1 1
  spline S786 degree 2 poles (-31.0332, -45.5895) (-31.7706, -44.8169) (-32.8241, -44.7642) knots 0 0 0 1 1 1
  line L797 (-32.8241, -44.7642) -> (-32.9997, -44.7642)
  spline S787 degree 2 poles (-32.9997, -44.7642) (-33.9303, -44.7642) (-34.6502, -45.3963) knots 0 0 0 1 1 1
  spline S788 degree 2 poles (-34.6502, -45.3963) (-35.4404, -46.1162) (-35.493, -47.1697) knots 0 0 0 1 1 1
  line L798 (-35.493, -47.1697) -> (-35.493, -47.3102)
  spline S789 degree 2 poles (-35.493, -47.3102) (-35.493, -49.5226) (-32.2623, -53.0694) knots 0 0 0 1 1 1
  spline S790 degree 2 poles (-32.2623, -53.0694) (-29.1017, -56.5811) (-29.1017, -59.8997) knots 0 0 0 1 1 1
  spline S791 degree 2 poles (-29.1017, -59.8997) (-29.1017, -60.0753) (-29.1193, -60.2508) knots 0 0 0 1 1 1
  spline S792 degree 2 poles (-29.1193, -60.2508) (-29.2246, -62.112) (-30.5942, -63.3587) knots 0 0 0 1 1 1
  spline S793 degree 2 poles (-30.5942, -63.3587) (-31.876, -64.5) (-33.5616, -64.5) knots 0 0 0 1 1 1
  line L799 (-33.5616, -64.5) -> (-33.8074, -64.5)
  spline S794 degree 2 poles (-33.8074, -64.5) (-35.6511, -64.3946) (-36.8802, -63.0251) knots 0 0 0 1 1 1
  spline S795 degree 2 poles (-0.9569, -44.4482) (-0.9569, -44.0443) (-0.3951, -43.5) (-0.0088, -43.5) knots 0 0 0 1 2 2 2
  spline S796 degree 2 poles (-0.0088, -43.5) (0.3951, -43.5) (0.9569, -44.0443) (0.9569, -44.4482) knots 0 0 0 1 2 2 2
  line L800 (0.9569, -44.4482) -> (0.9569, -63.5518)
  spline S797 degree 2 poles (0.9569, -63.5518) (0.9569, -63.9381) (0.3951, -64.5) (-0.0088, -64.5) knots 0 0 0 1 2 2 2
  spline S798 degree 2 poles (-0.0088, -64.5) (-0.3951, -64.5) (-0.9569, -63.9381) (-0.9569, -63.5518) knots 0 0 0 1 2 2 2
  line L801 (-0.9569, -63.5518) -> (-0.9569, -44.4482)
  spline S799 degree 2 poles (29.7865, -63.0251) (29.488, -62.6739) (29.488, -62.2701) knots 0 0 0 1 1 1
  spline S800 degree 2 poles (29.488, -62.2701) (29.5231, -61.8662) (29.8041, -61.6028) knots 0 0 0 1 1 1
  spline S801 degree 2 poles (29.8041, -61.6028) (30.0674, -61.357) (30.4889, -61.357) knots 0 0 0 1 1 1
  spline S802 degree 2 poles (30.4889, -61.357) (30.8751, -61.3921) (31.2088, -61.7258) knots 0 0 0 1 1 1
  spline S803 degree 2 poles (31.2088, -61.7258) (31.9111, -62.5159) (32.9646, -62.5686) knots 0 0 0 1 1 1
  line L802 (32.9646, -62.5686) -> (33.0875, -62.5686)
  spline S804 degree 2 poles (33.0875, -62.5686) (34.0708, -62.5686) (34.7907, -61.9013) knots 0 0 0 1 1 1
  spline S805 degree 2 poles (34.7907, -61.9013) (35.5808, -61.199) (35.6335, -60.163) knots 0 0 0 1 1 1
  line L803 (35.6335, -60.163) -> (35.6335, -59.9523)
  spline S806 degree 2 poles (35.6335, -59.9523) (35.6335, -57.3186) (32.4378, -53.7893) knots 0 0 0 1 1 1
  spline S807 degree 2 poles (32.4378, -53.7893) (29.2598, -50.2776) (29.2598, -47.3278) knots 0 0 0 1 1 1
  line L804 (29.2598, -47.3278) -> (29.2598, -47.0644)
  spline S808 degree 2 poles (29.2598, -47.0644) (29.3651, -45.2032) (30.7347, -43.9741) knots 0 0 0 1 1 1
  spline S809 degree 2 poles (30.7347, -43.9741) (32.0164, -42.8328) (33.6845, -42.8328) knots 0 0 0 1 1 1
  line L805 (33.6845, -42.8328) -> (33.9479, -42.8328)
  spline S810 degree 2 poles (33.9479, -42.8328) (35.8091, -42.9381) (37.0206, -44.3077) knots 0 0 0 1 1 1
  spline S811 degree 2 poles (37.0206, -44.3077) (37.3367, -44.6589) (37.3367, -45.0452) knots 0 0 0 1 1 1
  spline S812 degree 2 poles (37.3367, -45.0452) (37.3016, -45.449) (37.0031, -45.7124) knots 0 0 0 1 1 1
  spline S813 degree 2 poles (37.0031, -45.7124) (36.7397, -45.9582) (36.371, -45.9582) knots 0 0 0 1 1 1
  spline S814 degree 2 poles (36.371, -45.9582) (35.932, -45.9406) (35.6335, -45.5895) knots 0 0 0 1 1 1
  spline S815 degree 2 poles (35.6335, -45.5895) (34.896, -44.8169) (33.8425, -44.7642) knots 0 0 0 1 1 1
  line L806 (33.8425, -44.7642) -> (33.6669, -44.7642)
  spline S816 degree 2 poles (33.6669, -44.7642) (32.7363, -44.7642) (32.0164, -45.3963) knots 0 0 0 1 1 1
  spline S817 degree 2 poles (32.0164, -45.3963) (31.2263, -46.1162) (31.1736, -47.1697) knots 0 0 0 1 1 1
  line L807 (31.1736, -47.1697) -> (31.1736, -47.3102)
  spline S818 degree 2 poles (31.1736, -47.3102) (31.1736, -49.5226) (34.4044, -53.0694) knots 0 0 0 1 1 1
  spline S819 degree 2 poles (34.4044, -53.0694) (37.5649, -56.5811) (37.5649, -59.8997) knots 0 0 0 1 1 1
  spline S820 degree 2 poles (37.5649, -59.8997) (37.5649, -60.0753) (37.5474, -60.2508) knots 0 0 0 1 1 1
  spline S821 degree 2 poles (37.5474, -60.2508) (37.442, -62.112) (36.0725, -63.3587) knots 0 0 0 1 1 1
  spline S822 degree 2 poles (36.0725, -63.3587) (34.7907, -64.5) (33.1051, -64.5) knots 0 0 0 1 1 1
  line L808 (33.1051, -64.5) -> (32.8593, -64.5)
  spline S823 degree 2 poles (32.8593, -64.5) (31.0156, -64.3946) (29.7865, -63.0251) knots 0 0 0 1 1 1
  spline S824 degree 2 poles (65.7097, -44.4482) (65.7097, -44.0443) (66.2716, -43.5) (66.6579, -43.5) knots 0 0 0 1 2 2 2
  spline S825 degree 2 poles (66.6579, -43.5) (67.0617, -43.5) (67.6236, -44.0443) (67.6236, -44.4482) knots 0 0 0 1 2 2 2
  line L809 (67.6236, -44.4482) -> (67.6236, -63.5518)
  spline S826 degree 2 poles (67.6236, -63.5518) (67.6236, -63.9381) (67.0617, -64.5) (66.6579, -64.5) knots 0 0 0 1 2 2 2
  spline S827 degree 2 poles (66.6579, -64.5) (66.2716, -64.5) (65.7097, -63.9381) (65.7097, -63.5518) knots 0 0 0 1 2 2 2
  line L810 (65.7097, -63.5518) -> (65.7097, -44.4482)
  spline S828 degree 2 poles (104.7847, -60.0577) (104.7847, -61.9013) (103.4678, -63.2007) knots 0 0 0 1 1 1
  spline S829 degree 2 poles (103.4678, -63.2007) (102.3089, -64.3946) (100.7111, -64.5) knots 0 0 0 1 1 1
  spline S830 degree 2 poles (100.7111, -64.5) (100.237, -64.5) (99.6927, -63.9381) (99.6927, -63.5518) knots 0 0 0 1 2 2 2
  spline S831 degree 2 poles (99.6927, -63.5518) (99.6927, -63.148) (99.9737, -62.8671) knots 0 0 0 1 1 1
  spline S832 degree 2 poles (99.9737, -62.8671) (100.2019, -62.6212) (100.5531, -62.5861) knots 0 0 0 1 1 1
  spline S833 degree 2 poles (100.5531, -62.5861) (101.4661, -62.5159) (102.1158, -61.8487) knots 0 0 0 1 1 1
  spline S834 degree 2 poles (102.1158, -61.8487) (102.8708, -61.1112) (102.8708, -60.0577) knots 0 0 0 1 1 1
  line L811 (102.8708, -60.0577) -> (102.8708, -57.4415)
  spline S835 degree 2 poles (102.8708, -57.4415) (102.8708, -56.4055) (102.1158, -55.6505) knots 0 0 0 1 1 1
  spline S836 degree 2 poles (102.1158, -55.6505) (101.5188, -55.036) (100.7111, -54.9306) knots 0 0 0 1 1 1
  spline S837 degree 2 poles (100.7111, -54.9306) (100.237, -54.9306) (99.9737, -54.6497) knots 0 0 0 1 1 1
  spline S838 degree 2 poles (99.9737, -54.6497) (99.6927, -54.3687) (99.6927, -53.9824) knots 0 0 0 1 1 1
  line L812 (99.6927, -53.9824) -> (99.6927, -53.9649)
  spline S839 degree 2 poles (99.6927, -53.9649) (99.6927, -53.561) (99.9737, -53.2801) knots 0 0 0 1 1 1
  spline S840 degree 2 poles (99.9737, -53.2801) (100.237, -52.9992) (100.7111, -52.9992) knots 0 0 0 1 1 1
  spline S841 degree 2 poles (100.7111, -52.9992) (101.5188, -52.8938) (102.1158, -52.2968) knots 0 0 0 1 1 1
  spline S842 degree 2 poles (102.1158, -52.2968) (102.8708, -51.5418) (102.8708, -50.4883) knots 0 0 0 1 1 1
  line L813 (102.8708, -50.4883) -> (102.8708, -47.9072)
  spline S843 degree 2 poles (102.8708, -47.9072) (102.8708, -46.8712) (102.1158, -46.1162) knots 0 0 0 1 1 1
  spline S844 degree 2 poles (102.1158, -46.1162) (101.4661, -45.4666) (100.5531, -45.3788) knots 0 0 0 1 1 1
  spline S845 degree 2 poles (100.5531, -45.3788) (100.2019, -45.3436) (99.9737, -45.0978) knots 0 0 0 1 1 1
  spline S846 degree 2 poles (99.9737, -45.0978) (99.6927, -44.8344) (99.6927, -44.4306) knots 0 0 0 1 1 1
  spline S847 degree 2 poles (99.6927, -44.4306) (99.6927, -44.0268) (100.237, -43.4824) (100.7111, -43.4824) knots 0 0 0 1 2 2 2
  spline S848 degree 2 poles (100.7111, -43.4824) (102.3089, -43.5878) (103.4678, -44.7642) knots 0 0 0 1 1 1
  spline S849 degree 2 poles (103.4678, -44.7642) (104.7847, -46.0635) (104.7847, -47.9072) knots 0 0 0 1 1 1
  line L814 (104.7847, -47.9072) -> (104.7847, -50.4883)
  spline S850 degree 2 poles (104.7847, -50.4883) (104.7847, -52.6656) (103.1166, -53.9824) knots 0 0 0 1 1 1
  spline S851 degree 2 poles (103.1166, -53.9824) (104.7847, -55.2818) (104.7847, -57.4415) knots 0 0 0 1 1 1
  line L815 (104.7847, -57.4415) -> (104.7847, -60.0577)
  spline S852 degree 2 poles (95.865, -44.4306) (95.865, -44.0268) (96.4268, -43.4824) (96.8131, -43.4824) knots 0 0 0 1 2 2 2
  spline S853 degree 2 poles (96.8131, -43.4824) (97.217, -43.4824) (97.7788, -44.0268) (97.7788, -44.4306) knots 0 0 0 1 2 2 2
  line L816 (97.7788, -44.4306) -> (97.7788, -63.5343)
  spline S854 degree 2 poles (97.7788, -63.5343) (97.7788, -63.9206) (97.217, -64.4824) (96.8131, -64.4824) knots 0 0 0 1 2 2 2
  spline S855 degree 2 poles (96.8131, -64.4824) (96.4268, -64.4824) (95.865, -63.9206) (95.865, -63.5343) knots 0 0 0 1 2 2 2
  line L817 (95.865, -63.5343) -> (95.865, -44.4306)
  spline S856 degree 2 poles (129.8392, -63.5518) (129.8392, -63.9381) (129.2773, -64.5) (128.8735, -64.5) knots 0 0 0 1 2 2 2
  spline S857 degree 2 poles (128.8735, -64.5) (128.4872, -64.5) (127.9253, -63.9381) (127.9253, -63.5518) knots 0 0 0 1 2 2 2